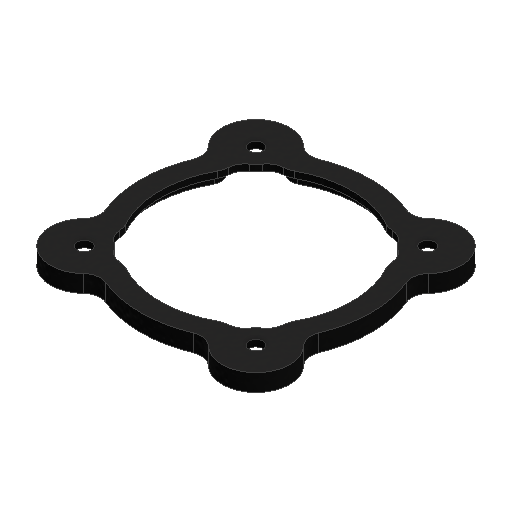
# Autodesk Inventor part: 3DP_ABS_Electronics_Colling_Fan_Grill_Honeycomb_Frame
Saved by Autodesk Inventor 2026.1 (Build 301233000, 233)
## iProperties
Created: 2017-07-01
Part Number: 3DP_ABS_Electronics_Colling_Fan_Grill_Honeycomb_Frame
Material: Ogólny
Document SubType Name: Modeling
Designer: Andrzej
Density: 1 g/cm^3
Appearance: Czarna
Author: Andrzej
Autodesk Inventor part; units mm, degrees
ref_plane "YZ Plane" through (0, 0, 0) normal (1, 0, 0) x (0, 1, 0)
ref_plane "XZ Plane" through (0, 0, 0) normal (0, 1, 0) x (-1, 0, 0)
ref_plane "XY Plane" through (0, 0, 0) normal (0, 0, 1) x (1, 0, 0)
sketch "Szkic1" plane through (0, 0, 0) normal (0, 0, 1) x (1, 0, 0)
  circle A0 centre (-23.62, 5.242) radius 1.5
  circle A1 centre (16.38, 5.242) radius 1.5
  circle A2 centre (16.38, 45.242) radius 1.5
  circle A3 centre (-23.62, 45.242) radius 1.5
  arc A4 (11.9508, 2.9221) -> (18.6999, 9.6712) centre (16.38, 5.242) ccw
  arc A5 (17.4572, 13.7635) -> (18.6999, 9.6712) centre (20.0918, 12.3287) ccw
  arc A6 (17.4572, 13.7635) -> (17.4572, 36.7204) centre (-3.62, 25.242) ccw
  arc A7 (18.6999, 40.8127) -> (17.4572, 36.7204) centre (20.0918, 38.1552) ccw
  arc A8 (18.6999, 40.8127) -> (11.9508, 47.5618) centre (16.38, 45.242) ccw
  arc A9 (7.8584, 46.3191) -> (11.9508, 47.5618) centre (9.2932, 48.9537) ccw
  arc A10 (7.8584, 46.3191) -> (-15.0984, 46.3191) centre (-3.62, 25.242) ccw
  arc A11 (-19.1907, 47.5618) -> (-15.0984, 46.3191) centre (-16.5332, 48.9537) ccw
  arc A12 (-19.1907, 47.5618) -> (-25.9399, 40.8127) centre (-23.62, 45.242) ccw
  arc A13 (-24.6971, 36.7204) -> (-25.9399, 40.8127) centre (-27.3318, 38.1552) ccw
  arc A14 (-24.6971, 36.7204) -> (-24.6971, 13.7635) centre (-3.62, 25.242) ccw
  arc A15 (-25.9399, 9.6712) -> (-24.6971, 13.7635) centre (-27.3318, 12.3287) ccw
  arc A16 (-25.9399, 9.6712) -> (-19.1907, 2.9221) centre (-23.62, 5.242) ccw
  arc A17 (-15.0984, 4.1648) -> (-19.1907, 2.9221) centre (-16.5332, 1.5302) ccw
  arc A18 (-15.0984, 4.1648) -> (7.8584, 4.1648) centre (-3.62, 25.242) ccw
  arc A19 (11.9508, 2.9221) -> (7.8584, 4.1648) centre (9.2932, 1.5302) ccw
  arc A20 (-18.8807, 47.7242) -> (-26.1022, 40.5027) centre (-23.62, 45.242) ccw
  arc A21 (-18.8807, 47.7242) -> (-15.2658, 46.6265) centre (-16.5332, 48.9537) ccw
  arc A22 (8.0258, 46.6265) -> (-15.2658, 46.6265) centre (-3.62, 25.242) ccw
  arc A23 (8.0258, 46.6265) -> (11.6407, 47.7242) centre (9.2932, 48.9537) ccw
  arc A24 (18.8623, 40.5027) -> (11.6407, 47.7242) centre (16.38, 45.242) ccw
  arc A25 (18.8623, 40.5027) -> (17.7645, 36.8878) centre (20.0918, 38.1552) ccw
  arc A26 (17.7645, 13.5962) -> (17.7645, 36.8878) centre (-3.62, 25.242) ccw
  arc A27 (17.7645, 13.5962) -> (18.8623, 9.9812) centre (20.0918, 12.3287) ccw
  arc A28 (11.6407, 2.7597) -> (18.8623, 9.9812) centre (16.38, 5.242) ccw
  arc A29 (11.6407, 2.7597) -> (8.0258, 3.8574) centre (9.2932, 1.5302) ccw
  arc A30 (-15.2658, 3.8574) -> (8.0258, 3.8574) centre (-3.62, 25.242) ccw
  arc A31 (-15.2658, 3.8574) -> (-18.8807, 2.7597) centre (-16.5332, 1.5302) ccw
  arc A32 (-26.1022, 9.9812) -> (-18.8807, 2.7597) centre (-23.62, 5.242) ccw
  arc A33 (-26.1022, 9.9812) -> (-25.0045, 13.5962) centre (-27.3318, 12.3287) ccw
  arc A34 (-25.0045, 36.8878) -> (-25.0045, 13.5962) centre (-3.62, 25.242) ccw
  arc A35 (-25.0045, 36.8878) -> (-26.1022, 40.5027) centre (-27.3318, 38.1552) ccw
  arc A36 (-16.5964, 48.748) -> (-27.126, 38.2184) centre (-23.62, 45.242) ccw
  arc A37 (9.3565, 48.748) -> (-16.5964, 48.748) centre (-3.62, 25.242) ccw
  arc A38 (19.8861, 38.2184) -> (9.3565, 48.748) centre (16.38, 45.242) ccw
  arc A39 (19.8861, 12.2655) -> (19.8861, 38.2184) centre (-3.62, 25.242) ccw
  arc A40 (9.3565, 1.7359) -> (19.8861, 12.2655) centre (16.38, 5.242) ccw
  arc A41 (-16.5964, 1.7359) -> (9.3565, 1.7359) centre (-3.62, 25.242) ccw
  arc A42 (-27.126, 12.2655) -> (-16.5964, 1.7359) centre (-23.62, 5.242) ccw
  arc A43 (-27.126, 38.2184) -> (-27.126, 12.2655) centre (-3.62, 25.242) ccw
  point P0 (0, 0)
  point P1 (0, 0)
  dimension "d0" = 0.35
  dimension "d1" = 2.5
  constraints: 80 point on circle, 44 centre point, 22 other
  measures "d0" radial gap between concentric circles of A13 A35
  measures "d1" radial gap between concentric circles of A20 A36
extrude "Wyciągnięcie proste1" add sketch "Szkic1" along normal blind 2.5 contours A37 A38 A39 A40 A41 A42 A43 A36
sketch "Szkic2" plane through (0, 0, 2.5) normal (0, 0, 1) x (1, 0, 0)
  arc A0 (-18.8807, 47.7242) -> (-15.2658, 46.6265) centre (-16.5332, 48.9537) ccw projected
  arc A1 (8.0258, 46.6265) -> (-15.2658, 46.6265) centre (-3.62, 25.242) ccw projected
  arc A2 (8.0258, 46.6265) -> (11.6407, 47.7242) centre (9.2932, 48.9537) ccw projected
  arc A3 (18.8623, 40.5027) -> (11.6407, 47.7242) centre (16.38, 45.242) ccw projected
  arc A4 (18.8623, 40.5027) -> (17.7645, 36.8878) centre (20.0918, 38.1552) ccw projected
  arc A5 (17.7645, 13.5962) -> (17.7645, 36.8878) centre (-3.62, 25.242) ccw projected
  arc A6 (17.7645, 13.5962) -> (18.8623, 9.9812) centre (20.0918, 12.3287) ccw projected
  arc A7 (11.6407, 2.7597) -> (18.8623, 9.9812) centre (16.38, 5.242) ccw projected
  arc A8 (11.6407, 2.7597) -> (8.0258, 3.8574) centre (9.2932, 1.5302) ccw projected
  arc A9 (-15.2658, 3.8574) -> (8.0258, 3.8574) centre (-3.62, 25.242) ccw projected
  arc A10 (-15.2658, 3.8574) -> (-18.8807, 2.7597) centre (-16.5332, 1.5302) ccw projected
  arc A11 (-26.1022, 9.9812) -> (-18.8807, 2.7597) centre (-23.62, 5.242) ccw projected
  arc A12 (-26.1022, 9.9812) -> (-25.0045, 13.5962) centre (-27.3318, 12.3287) ccw projected
  arc A13 (-25.0045, 36.8878) -> (-25.0045, 13.5962) centre (-3.62, 25.242) ccw projected
  arc A14 (-25.0045, 36.8878) -> (-26.1022, 40.5027) centre (-27.3318, 38.1552) ccw projected
  arc A15 (-18.8807, 47.7242) -> (-26.1022, 40.5027) centre (-23.62, 45.242) ccw projected
  arc A16 (-16.5964, 48.748) -> (-27.126, 38.2184) centre (-23.62, 45.242) ccw projected
  arc A17 (-27.126, 38.2184) -> (-27.126, 12.2655) centre (-3.62, 25.242) ccw projected
  arc A18 (-27.126, 12.2655) -> (-16.5964, 1.7359) centre (-23.62, 5.242) ccw projected
  arc A19 (-16.5964, 1.7359) -> (9.3565, 1.7359) centre (-3.62, 25.242) ccw projected
  arc A20 (9.3565, 1.7359) -> (19.8861, 12.2655) centre (16.38, 5.242) ccw projected
  arc A21 (19.8861, 12.2655) -> (19.8861, 38.2184) centre (-3.62, 25.242) ccw projected
  arc A22 (19.8861, 38.2184) -> (9.3565, 48.748) centre (16.38, 45.242) ccw projected
  arc A23 (9.3565, 48.748) -> (-16.5964, 48.748) centre (-3.62, 25.242) ccw projected
  arc A24 (-25.1743, 8.2095) -> (-23.2481, 14.5527) centre (-27.3318, 12.3287) ccw
  arc A25 (-25.1743, 8.2095) -> (-20.6524, 3.6876) centre (-23.62, 5.242) ccw
  arc A26 (-14.3093, 5.6139) -> (-20.6524, 3.6876) centre (-16.5332, 1.5302) ccw
  arc A27 (-14.3093, 5.6139) -> (7.0693, 5.6139) centre (-3.62, 25.242) ccw
  arc A28 (13.4124, 3.6876) -> (7.0693, 5.6139) centre (9.2932, 1.5302) ccw
  arc A29 (13.4124, 3.6876) -> (17.9343, 8.2095) centre (16.38, 5.242) ccw
  arc A30 (16.0081, 14.5527) -> (17.9343, 8.2095) centre (20.0918, 12.3287) ccw
  arc A31 (16.0081, 14.5527) -> (16.0081, 35.9312) centre (-3.62, 25.242) ccw
  arc A32 (17.9343, 42.2744) -> (16.0081, 35.9312) centre (20.0918, 38.1552) ccw
  arc A33 (17.9343, 42.2744) -> (13.4124, 46.7963) centre (16.38, 45.242) ccw
  arc A34 (7.0693, 44.87) -> (13.4124, 46.7963) centre (9.2932, 48.9537) ccw
  arc A35 (7.0693, 44.87) -> (-14.3093, 44.87) centre (-3.62, 25.242) ccw
  arc A36 (-20.6524, 46.7963) -> (-14.3093, 44.87) centre (-16.5332, 48.9537) ccw
  arc A37 (-20.6524, 46.7963) -> (-25.1743, 42.2744) centre (-23.62, 45.242) ccw
  arc A38 (-23.2481, 35.9312) -> (-25.1743, 42.2744) centre (-27.3318, 38.1552) ccw
  arc A39 (-23.2481, 35.9312) -> (-23.2481, 14.5527) centre (-3.62, 25.242) ccw
  arc A40 (-18.6389, 5.6761) -> (-23.1859, 10.2231) centre (-23.62, 5.242) ccw
  arc A41 (15.9459, 10.2231) -> (11.3989, 5.6761) centre (16.38, 5.242) ccw
  arc A42 (11.3989, 44.8078) -> (15.9459, 40.2608) centre (16.38, 45.242) ccw
  arc A43 (-23.1859, 40.2608) -> (-18.6389, 44.8078) centre (-23.62, 45.242) ccw
  point P0 (0, 0)
  dimension "d4" = 2
  dimension "d5" = 10
  dimension "d6" = 10
  dimension "d7" = 10
  dimension "d8" = 10
  constraints: 48 point on circle, 20 centre point, 8 coincident, 15 other
  measures "d4" radial gap between concentric circles of A13 A39
  measures "d5" diameter of A40
  measures "d6" diameter of A41
  measures "d7" diameter of A42
  measures "d8" diameter of A43
extrude "Wyciągnięcie proste2" add sketch "Szkic2" along normal blind 1.5 contours A0 A1 A2 A3 A4 A5 A6 A7 A8 A9 A10 A11 A12 A13 A14 A15 | A23 A22 A21 A20 A19 A18 A17 A16 | A24 A40 A26 A25 | A38 A37 A36 A43 | A41 A30 A29 A28 | A34 A33 A32 A42
fillet "Zaokrąglenie1" radius 4 24 edges at (-18.6389, 44.8078, 3.25) (-23.1859, 40.2608, 3.25) (11.3989, 44.8078, 3.25) (15.9459, 40.2608, 3.25) (15.9459, 10.2231, 3.25) (11.3989, 5.6761, 3.25) (-18.6389, 5.6761, 3.25) (-23.1859, 10.2231, 3.25) (-27.126, 38.2184, 1.25) (-27.126, 38.2184, 3.25) (-27.126, 12.2655, 1.25) (-27.126, 12.2655, 3.25) (-16.5964, 48.748, 1.25) (-16.5964, 48.748, 3.25) (9.3565, 48.748, 1.25) (9.3565, 48.748, 3.25) (19.8861, 38.2184, 1.25) (19.8861, 38.2184, 3.25) (19.8861, 12.2655, 1.25) (19.8861, 12.2655, 3.25) (9.3565, 1.7359, 1.25) (9.3565, 1.7359, 3.25) (-16.5964, 1.7359, 1.25) (-16.5964, 1.7359, 3.25)
hole "Otwór1" at (16.38, 5.242, 2.5) at (-23.62, 5.242, 2.5) at (-23.62, 45.242, 2.5) at (16.38, 45.242, 2.5) direction (0, 0, 1) diameter 3.3 end through all
